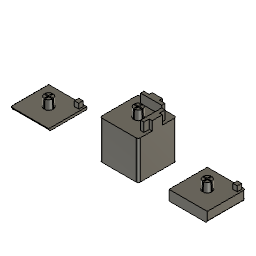
ProfilendkappenUNDFueße (Autodesk Fusion 360 design; units mm, degrees)
part number: 2025-10-27-17-13-30-402
Autodesk Fusion 360 part; units mm, degrees
note: some values were not read from the file. Chosen so that the rebuilt part matches the saved one: which bodies a step acts on; which face or edge a step refers to; which pieces of a blend or face edit are solid.
sketch "Skizze1" plane through (0, 0, 0) normal (0, 0, 1) x (1, 0, 0)
  line L0 (0, 0) -> (30, 0)
  line L1 (30, 0) -> (30, 30)
  line L2 (30, 30) -> (0, 30)
  line L3 (0, 30) -> (0, 0)
  dimension "d1" = 30
  dimension "d2" = 30
  constraint horizontal L0
  constraint vertical L1
  constraint horizontal L2
  constraint vertical L3
  constraint coincident L0.start L3.end
  measures "d1" distance of L0.start L0.end
  measures "d2" distance of L0.start L2.end
extrude "Extrusion1" add sketch "Skizze1" along normal blind 2 makes body 1
fillet "Abrundung1" radius 1.5 1 edges at (0, 0, 1) on bodies 1
fillet "Abrundung2" radius 1.5 3 edges at (0, 15.75, 0) (0.4393, 0.4393, 0) (15.75, 0, 0) on bodies 1
sketch "Skizze2" plane through (0, 0, 2) normal (0, 0, 1) x (-1, 0, 0)
  line L0 (0, -30) -> (0, -1.5)
  arc A0 (0, -1.5) -> (-1.5, 0) centre (-1.5, -1.5) ccw
  line L1 (-1.5, 0) -> (-30, 0)
  line L2 (-30, 0) -> (-30, -30)
  line L3 (-30, -30) -> (0, -30)
  line L4 (0, 0) -> (-13, 0)
  line L5 (0, 0) -> (-1.5, 0)
  line L6 (-1.5, 0) -> (-1.5, -1.5)
  line L7 (-1.5, -1.5) -> (0, -1.5)
  line L8 (0, -1.5) -> (0, 0)
  line L9 (-1.5, -1.5) -> (-5, -1.5)
  line L10 (-5, -1.5) -> (-5, -5)
  line L11 (-5, -5) -> (-1.5, -5)
  line L12 (-1.5, -5) -> (-1.5, -1.5)
  line L13 (0, -30) -> (-1.5, -30)
  line L14 (-1.5, -30) -> (-1.5, -28.5)
  line L15 (-1.5, -28.5) -> (0, -28.5)
  line L16 (0, -28.5) -> (0, -30)
  line L17 (-1.5, -28.5) -> (-5, -28.5)
  line L18 (-5, -28.5) -> (-5, -25)
  line L19 (-5, -25) -> (-1.5, -25)
  line L20 (-1.5, -25) -> (-1.5, -28.5)
  line L21 (-30, -30) -> (-28.5, -30)
  line L22 (-28.5, -30) -> (-28.5, -28.5)
  line L23 (-28.5, -28.5) -> (-30, -28.5)
  line L24 (-30, -28.5) -> (-30, -30)
  line L25 (-28.5, -28.5) -> (-25, -28.5)
  line L26 (-25, -28.5) -> (-25, -25)
  line L27 (-25, -25) -> (-28.5, -25)
  line L28 (-28.5, -25) -> (-28.5, -28.5)
  line L29 (-30, 0) -> (-28.5, 0)
  line L30 (-28.5, 0) -> (-28.5, -1.5)
  line L31 (-28.5, -1.5) -> (-30, -1.5)
  line L32 (-30, -1.5) -> (-30, 0)
  line L33 (-28.5, -1.5) -> (-25, -1.5)
  line L34 (-25, -1.5) -> (-25, -5)
  line L35 (-25, -5) -> (-28.5, -5)
  line L36 (-28.5, -5) -> (-28.5, -1.5)
  line L37 (0, 0) -> (-15, 0)
  line L38 (-15, 0) -> (-15, -15)
  line L39 (-15, -15) -> (0, -15)
  line L40 (0, -15) -> (0, 0)
  circle A1 centre (-15, -15) radius 3.575
  line L41 (-14.6, -18.6) -> (-15.4, -18.6)
  line L42 (-15.4, -18.6) -> (-15.4, -11.4)
  line L43 (-15.4, -11.4) -> (-14.6, -11.4)
  line L44 (-14.6, -11.4) -> (-14.6, -18.6)
  line L45 (-14.6, -18.6) -> (-15.4, -11.4) construction
  line L46 (-15.4, -18.6) -> (-14.6, -11.4) construction
  line L47 (-18.6, -15.4) -> (-11.4, -15.4)
  line L48 (-11.4, -15.4) -> (-11.4, -14.6)
  line L49 (-11.4, -14.6) -> (-18.6, -14.6)
  line L50 (-18.6, -14.6) -> (-18.6, -15.4)
  line L51 (-18.6, -15.4) -> (-11.4, -14.6) construction
  line L52 (-11.4, -15.4) -> (-18.6, -14.6) construction
  point P0 (-15, -15)
  point P1 (-15, -15)
  dimension "d10" = 1.5
  dimension "d11" = 1.5
  dimension "d12" = 3.5
  dimension "d13" = 3.5
  dimension "d14" = 1.5
  dimension "d15" = 1.5
  dimension "d16" = 3.5
  dimension "d17" = 3.5
  dimension "d18" = 1.5
  dimension "d19" = 1.5
  dimension "d20" = 3.5
  dimension "d21" = 3.5
  dimension "d22" = 1.5
  dimension "d23" = 1.5
  dimension "d24" = 3.5
  dimension "d25" = 3.5
  dimension "d28" = 15
  dimension "d29" = 15
  dimension "d30" = 7.15
  dimension "d31" = 0.8
  dimension "d32" = 0.8
  dimension "d33" = 7.2
  dimension "d34" = 7.2
  constraint coincident L4.start L5.start
  constraint parallel L1 L4
  constraint horizontal L5
  constraint vertical L6
  constraint horizontal L7
  constraint vertical L8
  constraint horizontal L9
  constraint vertical L10
  constraint horizontal L11
  constraint vertical L12
  constraint horizontal L13
  constraint vertical L14
  constraint horizontal L15
  constraint vertical L16
  constraint horizontal L17
  constraint vertical L18
  constraint horizontal L19
  constraint vertical L20
  constraint horizontal L21
  constraint vertical L22
  constraint horizontal L23
  constraint vertical L24
  constraint horizontal L25
  constraint vertical L26
  constraint horizontal L27
  constraint vertical L28
  constraint horizontal L29
  constraint vertical L30
  constraint horizontal L31
  constraint vertical L32
  constraint horizontal L33
  constraint vertical L34
  constraint horizontal L35
  constraint vertical L36
  constraint horizontal L37
  constraint vertical L38
  constraint horizontal L39
  constraint vertical L40
  constraint coincident P1 P0
  constraint horizontal L41
  constraint perpendicular L41 L42
  constraint parallel L41 L43
  constraint parallel L42 L44
  constraint coincident L45 P1
  constraint coincident L46 P1
  constraint horizontal L47
  constraint perpendicular L47 L48
  constraint parallel L47 L49
  constraint parallel L48 L50
  constraint coincident L51 P1
  constraint coincident L52 P1
  measures "d10" distance of L4.start A0.end
  measures "d11" distance of L4.start L0.end
  measures "d12" distance of A0.centre L9.end
  measures "d13" distance of A0.centre L11.end
  measures "d14" distance of L0.start L13.end
  measures "d15" distance of L0.start L15.end
  measures "d16" distance of L14.end L17.end
  measures "d17" distance of L14.end L19.end
  measures "d18" distance of L2.end L21.end
  measures "d19" distance of L2.end L23.end
  measures "d20" distance of L22.end L25.end
  measures "d21" distance of L22.end L27.end
  measures "d22" distance of L1.end L29.end
  measures "d23" distance of L1.end L31.end
  measures "d24" distance of L30.end L33.end
  measures "d25" distance of L30.end L35.end
  measures "d28" distance of L4.start L37.end
  measures "d29" distance of L4.start L39.end
  measures "d30" diameter of A1
  measures "d31" distance of L42.end L43.end
  measures "d32" distance of L47.end L48.end
  measures "d33" distance of L48 L50
  measures "d34" distance of L43.end L41
extrude "Extrusion3" add sketch "Skizze2" along normal blind 7 contours A1 L44 L49 | A1 L44 L47 | A1 L42 L47 | A1 L42 L49 bodies 1
chamfer "Fase1" distance 0.2 distance2 7 1 edges at (17.5279, 12.4721, 9) measured on face at (16.8139, 13.1861, 9) on bodies 1
chamfer "Fase2" distance 0.2 distance2 7 3 edges at (12.4721, 12.4721, 9) (12.4721, 17.5279, 9) (17.5279, 17.5279, 9) measured on face at (13.1861, 13.1861, 9) measured on face at (13.1861, 16.8139, 9) measured on face at (16.8139, 16.8139, 9) on bodies 1
extrude "Extrusion4" add sketch "Skizze2" along normal blind 4 contours L25 L26 L27 L28 bodies 1
copy_body "Körper kopieren/einfügen1" bodies 1 makes body 2
move_body "Verschieben1" bodies 2 to x (1, 0, 0) y (0, 1, 0) z (0, 0, 1) at (70, 0, 28)
sketch "Skizze3" plane through (0, 0, 30) normal (0, 0, 1) x (-1, 0, 0)
  line L0 (-98.5, -25) -> (-95, -25)
  line L1 (-95, -25) -> (-95, -28.5)
  line L2 (-95, -28.5) -> (-98.5, -28.5)
  line L3 (-98.5, -28.5) -> (-98.5, -25)
  line L4 (-85.4, -14.6) -> (-88.5526, -14.6)
  arc A0 (-85.4, -11.4474) -> (-88.5526, -14.6) centre (-85, -15) ccw
  line L5 (-85.4, -11.4474) -> (-85.4, -14.6)
  line L6 (-84.6, -15.4) -> (-81.4474, -15.4)
  arc A1 (-84.6, -18.5526) -> (-81.4474, -15.4) centre (-85, -15) ccw
  line L7 (-84.6, -18.5526) -> (-84.6, -15.4)
  line L8 (-88.5526, -15.4) -> (-85.4, -15.4)
  line L9 (-85.4, -15.4) -> (-85.4, -18.5526)
  arc A2 (-88.5526, -15.4) -> (-85.4, -18.5526) centre (-85, -15) ccw
  line L10 (-81.4474, -14.6) -> (-84.6, -14.6)
  line L11 (-84.6, -14.6) -> (-84.6, -11.4474)
  arc A3 (-81.4474, -14.6) -> (-84.6, -11.4474) centre (-85, -15) ccw
  arc A4 (-70, -1.5) -> (-71.5, 0) centre (-71.5, -1.5) ccw
  line L12 (-71.5, 0) -> (-100, 0)
  line L13 (-100, 0) -> (-100, -30)
  line L14 (-100, -30) -> (-70, -30)
  line L15 (-70, -30) -> (-70, -1.5)
  line L16 (-100, -30) -> (-70, -30)
  line L17 (-70, -30) -> (-70, 0)
  line L18 (-70, 0) -> (-100, 0)
  line L19 (-100, 0) -> (-100, -30)
  constraint horizontal L16
  constraint vertical L17
  constraint horizontal L18
  constraint vertical L19
  constraint coincident L13.end L14.start
extrude "Extrusion5" add sketch "Skizze3" against normal blind 30 contours A4 L12 L13 L14 L15 L16 L17 L18 L19 bodies 2
extrude "Extrusion6" add 5 faces at (86.8139, 13.1861, 28) (83.1861, 13.1861, 28) (83.1861, 16.8139, 28) (86.8139, 16.8139, 28) (96.1667, 27.3333, 28) along direction (0, 0, -1) blind 28 on bodies 2 bodies 2
fillet "Abrundung3" radius 1.5 3 edges at (70, 30, 15) (100, 30, 15) (100, 0, 15) on bodies 2
copy_body "Körper kopieren/einfügen2" bodies 2 makes body 3
move_body "Verschieben2" bodies 3 to x (1, 0, 0) y (0, 1, 0) z (0, 0, 1) at (54, 0, 0)
split "Teilen1" by plane through (124, 0, 30) normal (0, 0, 1) bodies 3 makes body 4 at (139.7105, 18.4522, 31.7681) makes body 5 at (135.5478, 14.2895, 31.7681) makes body 6 at (135.5478, 15.7105, 31.7681) makes body 7 at (139.7105, 11.5478, 31.7681) makes body 8 at (150.1667, 28.5, 32.6667)
extrude "Extrusion7" cut 6 faces at (127.8158, 15.1333, 30) (137.1861, 13.1861, 30) (140.8139, 13.1861, 30) (137.1861, 16.8139, 30) (140.8139, 16.8139, 30) (151.3333, 27.3333, 30) along direction (0, 0, -1) blind 25 on bodies 3 bodies 3
move_body "Verschieben3" bodies 5 4 6 7 8 to x (1, 0, 0) y (0, 1, 0) z (0, 0, 1) at (0, 0, -25)
delete_face "Fläche löschen1" 1 faces at (124.4144, 0.4649, 1.6667) on bodies 3
delete_face "Fläche löschen2" 1 faces at (124.6299, 29.7219, 3.3333) on bodies 3
delete_face "Fläche löschen3" 1 faces at (153.0575, 0.1074, 1.6667) on bodies 3
fillet "Abrundung4" radius 1.5 3 edges at (138.25, 30, 0) (153.5607, 29.5607, 0) (154, 14.25, 0) on bodies 3
move_body "Verschieben4" bodies 7 4 6 5 8 to x (1, 0, 0) y (0, 1, 0) z (0, 0, 1) at (0, 0, 3)
extrude "Extrusion8" add 1 faces at (133.5, 20, 5) along direction (0, 0, 1) blind 3 on bodies 3 bodies 3 4 5 6 7 8
delete_face "Fläche löschen4" 1 faces at (96.1667, 25, 31.3333) on bodies 2
sketch "Skizze4" plane through (0, 0, 30) normal (0, 0, 1) x (-1, 0, 0)
  line L0 (-85.4, -14.6) -> (-88.5526, -14.6)
  arc A0 (-85.4, -11.4474) -> (-88.5526, -14.6) centre (-85, -15) ccw
  line L1 (-85.4, -11.4474) -> (-85.4, -14.6)
  line L2 (-84.6, -15.4) -> (-81.4474, -15.4)
  arc A1 (-84.6, -18.5526) -> (-81.4474, -15.4) centre (-85, -15) ccw
  line L3 (-84.6, -18.5526) -> (-84.6, -15.4)
  line L4 (-88.5526, -15.4) -> (-85.4, -15.4)
  line L5 (-85.4, -15.4) -> (-85.4, -18.5526)
  arc A2 (-88.5526, -15.4) -> (-85.4, -18.5526) centre (-85, -15) ccw
  line L6 (-81.4474, -14.6) -> (-84.6, -14.6)
  line L7 (-84.6, -14.6) -> (-84.6, -11.4474)
  arc A3 (-81.4474, -14.6) -> (-84.6, -11.4474) centre (-85, -15) ccw
  arc A4 (-98.5, 0) -> (-100, -1.5) centre (-98.5, -1.5) ccw
  line L8 (-100, -1.5) -> (-100, -28.5)
  arc A5 (-100, -28.5) -> (-98.5, -30) centre (-98.5, -28.5) ccw
  line L9 (-98.5, -30) -> (-71.5, -30)
  arc A6 (-71.5, -30) -> (-70, -28.5) centre (-71.5, -28.5) ccw
  line L10 (-70, -28.5) -> (-70, -1.5)
  arc A7 (-70, -1.5) -> (-71.5, 0) centre (-71.5, -1.5) ccw
  line L11 (-71.5, 0) -> (-98.5, 0)
  line L12 (-100, -15) -> (-100, -19)
  line L13 (-100, -19) -> (-97.7, -19)
  line L14 (-97.7, -19) -> (-97.7, -23.3)
  line L15 (-97.7, -23.3) -> (-95.1, -23.3)
  line L16 (-100, -10.8) -> (-100, -15)
  line L17 (-100, -15) -> (-100, -11)
  line L18 (-100, -11) -> (-97.7, -11)
  line L19 (-97.7, -11) -> (-97.7, -6.7)
  line L20 (-97.7, -6.7) -> (-95.1, -6.7)
  line L21 (-95.1, -6.7) -> (-95.1, -23.3)
  line L22 (-85, -30) -> (-89, -30)
  line L23 (-89, -30) -> (-89, -27.7)
  line L24 (-89, -27.7) -> (-93.3, -27.7)
  line L25 (-93.3, -27.7) -> (-93.3, -25.1)
  line L26 (-93.3, -25.1) -> (-76.7, -25.1)
  line L27 (-76.7, -25.1) -> (-76.7, -27.7)
  line L28 (-76.7, -27.7) -> (-81, -27.7)
  line L29 (-81, -27.7) -> (-81, -30)
  line L30 (-81, -30) -> (-85, -30)
  dimension "d55" = 4
  dimension "d56" = 2.3
  dimension "d57" = 4.3
  dimension "d58" = 2.6
  dimension "d62" = 4.3
  dimension "d63" = 4
  dimension "d64" = 2.3
  dimension "d65" = 4.3
  dimension "d66" = 2.6
  dimension "d67" = 16.6
  dimension "d68" = 2.6
  dimension "d69" = 4.3
  constraint midpoint L8 L12.start
  constraint parallel L8 L12
  constraint perpendicular L12 L13
  constraint perpendicular L13 L14
  constraint perpendicular L14 L15
  constraint coincident L8 L16.start
  constraint coincident L16 L17.end
  constraint perpendicular L18 L19
  constraint perpendicular L19 L20
  constraint perpendicular L15 L21
  constraint midpoint L9 L22.start
  constraint perpendicular L21 L22
  constraint perpendicular L22 L23
  constraint perpendicular L23 L24
  constraint perpendicular L24 L25
  constraint perpendicular L25 L26
  constraint perpendicular L26 L27
  constraint perpendicular L27 L28
  constraint coincident L9 L29.end
  constraint perpendicular L9 L29
  measures "d55" distance of L12.start L12.end
  measures "d56" distance of L12.end L13.end
  measures "d57" distance of L13.end L14.end
  measures "d58" distance of L14.end L15.end
  measures "d62" distance of L18.end L19.end
  measures "d63" distance of L22.start L22.end
  measures "d64" distance of L22.end L23.end
  measures "d65" distance of L23.end L24.end
  measures "d66" distance of L24.end L25.end
  measures "d67" distance of L25.end L26.end
  measures "d68" distance of L26.end L27.end
  measures "d69" distance of L27.end L28.end
extrude "Extrusion9" add sketch "Skizze4" along normal blind 7 contours L8 L12 L13 L14 L15 L16 L17 L18 L19 L20 L21 | L9 L22 L23 L24 L25 L26 L27 L28 L29 L30 bodies 2
